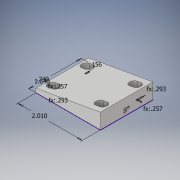
# Autodesk Inventor part: shim 10 Deg
Saved by Autodesk Inventor 2018 (Build 220112000, 112)
## iProperties
Created: 2018-03-27
Part Number: shim 10 Deg
Material: Generic
Document SubType Name: Modeling
Designer: prakh
Density: 1 g/cm^3
Appearance: Default
Author: prakh
Autodesk Inventor part; units mm, degrees
ref_plane "YZ Plane" through (0, 0, 0) normal (1, 0, 0) x (0, 1, 0)
ref_plane "XZ Plane" through (0, 0, 0) normal (0, 1, 0) x (-1, 0, 0)
ref_plane "XY Plane" through (0, 0, 0) normal (0, 0, 1) x (1, 0, 0)
sketch "Sketch1" plane through (0, 0, 0) normal (0, 1, 0) x (-1, 0, 0)
  line L0 (25.527, 20.828) -> (-25.527, 20.828)
  line L1 (-25.527, 20.828) -> (-25.527, -20.828)
  line L2 (-25.527, -20.828) -> (25.527, -20.828)
  line L3 (25.527, -20.828) -> (25.527, 20.828)
  circle A0 centre (18.9992, 13.3858) radius 1.9837
  circle A1 centre (18.9992, -13.3858) radius 1.9837
  circle A2 centre (-18.9992, -13.3858) radius 1.9837
  circle A3 centre (-18.9992, 13.3858) radius 1.9837
  circle A4 centre (18.9992, 13.3858) radius 3.048 construction
  point P0 (0, 0)
  point P1 (25.527, 0)
  point P2 (0, -20.828)
  dimension "d0" = 3.9675
  dimension "d1" = 41.656
  dimension "d2" = 51.054
  dimension "d3" = 6.096
  dimension "d4" = 7.4422
  dimension "d5" = 6.5278
  dimension "d6" = 7.4422
  dimension "d7" = 6.5278
  constraints: 8 end point, 5 centre point, 3 equal radius, 3 horizontal alignment, 3 vertical alignment, 2 midpoint, 2 parallel, 1 coincident, 1 horizontal, 1 perpendicular
  measures "d0" diameter of A1
  measures "d1" distance of L2.end L0.start
  measures "d2" distance of L0.start L0.end
  measures "d3" diameter of A4
  measures "d4" distance from line of L0 A4.centre
  measures "d5" distance from line of A4.centre L3
  measures "d6" distance from line of L2 A2.centre
  measures "d7" distance from line of A2.centre L1
sketch "Sketch10" plane through (0, 0, 0) normal (0, 0, 1) x (1, 0, 0)
  line L0 (-25.527, 0) -> (25.527, 0)
  line L1 (25.527, 0) -> (25.527, 12.1772)
  line L2 (-25.527, 0) -> (-25.527, 3.175)
  line L3 (-25.527, 3.175) -> (25.527, 12.1772)
  point P0 (0, 0)
  dimension "d61" = 10
  dimension "d62" = 3.175
  constraints: 8 end point, 1 horizontal, 1 perpendicular, 1 vertical
  measures "d61" angle of L0 L3
  measures "d62" distance of L0.start L2.end
extrude "Extrusion8" add sketch "Sketch10" along normal mid plane 41.656
sketch "Sketch11" plane through (-25.527, 0, 20.828) normal (0, -1, 0) x (1, 0, 0)
  line L0 (46.1137, -7.4422) -> (42.9387, -7.4422) construction
  line L1 (46.1137, -4.3942) -> (42.9387, -4.3942)
  line L2 (42.9387, -10.4902) -> (46.1137, -10.4902)
  arc A0 (46.1137, -10.4902) -> (46.1137, -4.3942) centre (46.1137, -7.4422) ccw
  arc A1 (42.9387, -4.3942) -> (42.9387, -10.4902) centre (42.9387, -7.4422) ccw
  line L3 (46.1137, -34.2138) -> (42.9387, -34.2138) construction
  line L4 (51.054, -41.656) -> (51.054, 0) projected
  line L5 (46.1137, -37.2618) -> (42.9387, -37.2618)
  line L6 (42.9387, -31.1658) -> (46.1137, -31.1658)
  arc A2 (46.1137, -37.2618) -> (46.1137, -31.1658) centre (46.1137, -34.2138) ccw
  arc A3 (42.9387, -31.1658) -> (42.9387, -37.2618) centre (42.9387, -34.2138) ccw
  line L7 (8.1153, -34.2138) -> (4.9403, -34.2138) construction
  line L8 (8.1153, -37.2618) -> (4.9403, -37.2618)
  line L9 (4.9403, -31.1658) -> (8.1153, -31.1658)
  arc A4 (8.1153, -37.2618) -> (8.1153, -31.1658) centre (8.1153, -34.2138) ccw
  arc A5 (4.9403, -31.1658) -> (4.9403, -37.2618) centre (4.9403, -34.2138) ccw
  line L10 (8.1153, -7.4422) -> (4.9403, -7.4422) construction
  line L11 (8.1153, -10.4902) -> (4.9403, -10.4902)
  line L12 (4.9403, -4.3942) -> (8.1153, -4.3942)
  arc A6 (8.1153, -10.4902) -> (8.1153, -4.3942) centre (8.1153, -7.4422) ccw
  arc A7 (4.9403, -4.3942) -> (4.9403, -10.4902) centre (4.9403, -7.4422) ccw
  point P0 (25.527, -20.828)
  point P1 (44.5262, -7.4422)
  point P2 (44.5262, -34.2138)
  point P3 (6.5278, -34.2138)
  point P4 (6.5278, -7.4422)
  point P5 (44.5262, -7.4422)
  point P6 (44.5262, -34.2138)
  point P7 (6.5278, -34.2138)
  point P8 (6.5278, -7.4422)
  point P9 (44.5262, -10.4902)
  point P10 (6.5278, -37.2618)
  dimension "d65" = 3.175
  dimension "d66" = 3.048
  constraints: 32 end point, 16 point on circle, 16 tangent, 8 centre point, 8 horizontal alignment, 6 midpoint, 6 vertical alignment, 4 parallel, 4 point on line, 3 equal radius, 1 collinear, 1 horizontal, 1 perpendicular
  measures "d65" distance of L3.start L3.end
  measures "d66" radius of A6
extrude "Extrusion9" cut sketch "Sketch11" against normal blind 41.656
sketch "Sketch13" plane through (25.527, 0, 20.828) normal (1, 0, 0) x (0, 0, -1)
  line L0 (41.656, 12.1772) -> (0, 12.1772) projected
  line L1 (0, 0) -> (0, 12.1772) projected
  line L2 (41.656, 0) -> (0, 0) projected
  line L3 (41.656, 12.1772) -> (41.656, 0) projected
  line L4 (25.4999, 2.032) -> (16.1561, 2.032)
  spline S0 degree 2 poles (20.8859, 3.1075) (20.8859, 2.8579) (20.7161, 2.436) (20.5488, 2.2841) knots 0 0 0 1 2 2 2
  spline S1 degree 2 poles (20.5488, 2.2841) (20.3816, 2.1323) (19.9236, 1.9651) (19.5891, 1.9651) knots 0 0 0 1 2 2 2
  spline S2 degree 2 poles (19.5891, 1.9651) (19.2341, 1.9677) (18.7246, 2.0835) (18.5574, 2.1581) knots 0 0 0 1 2 2 2
  line L5 (18.5574, 2.1581) -> (18.5574, 2.8502)
  line L6 (18.5574, 2.8502) -> (18.6294, 2.8502)
  spline S3 degree 2 poles (18.6294, 2.8502) (18.6912, 2.8167) (18.8404, 2.7293) (18.9613, 2.683) knots 0 0 0 1 2 2 2
  spline S4 degree 2 poles (18.9613, 2.683) (19.0745, 2.6392) (19.3087, 2.58) (19.4502, 2.58) knots 0 0 0 1 2 2 2
  spline S5 degree 2 poles (19.4502, 2.58) (19.5737, 2.58) (19.8619, 2.6418) (19.9493, 2.7241) knots 0 0 0 1 2 2 2
  spline S6 degree 2 poles (19.9493, 2.7241) (20.0137, 2.7884) (20.0857, 2.9454) (20.0857, 3.0766) knots 0 0 0 1 2 2 2
  spline S7 degree 2 poles (20.0857, 3.0766) (20.0857, 3.1898) (19.9931, 3.3493) (19.9185, 3.3982) knots 0 0 0 1 2 2 2
  spline S8 degree 2 poles (19.9185, 3.3982) (19.8104, 3.4703) (19.5017, 3.5114) (19.391, 3.5114) knots 0 0 0 1 2 2 2
  spline S9 degree 2 poles (19.391, 3.5114) (19.2161, 3.5114) (18.8841, 3.4548) (18.7632, 3.424) knots 0 0 0 1 2 2 2
  line L7 (18.7632, 3.424) -> (18.6938, 3.424)
  line L8 (18.6938, 3.424) -> (18.6938, 5.207)
  line L9 (18.6938, 5.207) -> (20.7984, 5.207)
  line L10 (20.7984, 5.207) -> (20.7984, 4.6075)
  line L11 (20.7984, 4.6075) -> (19.4476, 4.6075)
  line L12 (19.4476, 4.6075) -> (19.4476, 4.0801)
  spline S10 degree 2 poles (19.4476, 4.0801) (19.5119, 4.0852) (19.6895, 4.0903) (19.7384, 4.0903) knots 0 0 0 1 2 2 2
  spline S11 degree 2 poles (19.7384, 4.0903) (19.9674, 4.0903) (20.3533, 3.9977) (20.5051, 3.9025) knots 0 0 0 1 2 2 2
  spline S12 degree 2 poles (20.5051, 3.9025) (20.6852, 3.7842) (20.8859, 3.3905) (20.8859, 3.1075) knots 0 0 0 1 2 2 2
  spline S13 degree 2 poles (23.0832, 4.4145) (23.0832, 4.0518) (22.5789, 3.5552) (22.2187, 3.5552) knots 0 0 0 1 2 2 2
  spline S14 degree 2 poles (22.2187, 3.5552) (21.8559, 3.5552) (21.3516, 4.0518) (21.3516, 4.4145) knots 0 0 0 1 2 2 2
  spline S15 degree 2 poles (21.3516, 4.4145) (21.3516, 4.7773) (21.8559, 5.2739) (22.2187, 5.2739) knots 0 0 0 1 2 2 2
  spline S16 degree 2 poles (22.2187, 5.2739) (22.5815, 5.2739) (23.0832, 4.7773) (23.0832, 4.4145) knots 0 0 0 1 2 2 2
  spline S17 degree 2 poles (22.6175, 4.4145) (22.6175, 4.5818) (22.3885, 4.8211) (22.2187, 4.8211) knots 0 0 0 1 2 2 2
  spline S18 degree 2 poles (22.2187, 4.8211) (22.0489, 4.8211) (21.8173, 4.5844) (21.8173, 4.4145) knots 0 0 0 1 2 2 2
  spline S19 degree 2 poles (21.8173, 4.4145) (21.8173, 4.2396) (22.0514, 4.008) (22.2187, 4.008) knots 0 0 0 1 2 2 2
  spline S20 degree 2 poles (22.2187, 4.008) (22.3885, 4.008) (22.6175, 4.2447) (22.6175, 4.4145) knots 0 0 0 1 2 2 2
  point P0 (20.828, 0)
  point P1 (20.828, 0)
  point P2 (20.828, 2.032)
  dimension "d69" = 2.032
  constraints: 2 end point, 2 horizontal, 2 midpoint, 1 vertical alignment
  measures "d69" distance between parallel lines of L2 L4
extrude "Extrusion10" cut sketch "Sketch13" against normal blind 0.381 contours S1 S2 L4 | L4 S2 L5 L6 S3 S4 S5 S6 S7 S8 S9 L7 L8 L9 L10 L11 L12 S10 S11 S12 S0 S1 | S13 S14 S15 S16
equation "\"d6\" = d4"
equation "\"d7\" = d5"
equation "\"d23\" = d22"
equation "\"d25\" = 0.5 * d24"
equation "\"d22\" = 3.175"
equation "\"d24\" = 4.7625"
body "Solid2"
